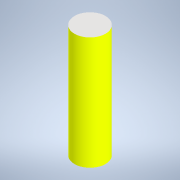
# Autodesk Inventor part: pieza2
Saved by Autodesk Inventor 2021 (Build 250183000, 183)
## iProperties
Created: 2023-05-09
Part Number: pieza2
Material: Generic
Document SubType Name: Modeling
Designer: assman
Density: 1 g/cm^3
Appearance: Default
Author: assman
Autodesk Inventor part; units mm, degrees
ref_plane "YZ Plane" through (0, 0, 0) normal (1, 0, 0) x (0, 1, 0)
ref_plane "XZ Plane" through (0, 0, 0) normal (0, 1, 0) x (-1, 0, 0)
ref_plane "XY Plane" through (0, 0, 0) normal (0, 0, 1) x (1, 0, 0)
sketch "Sketch1" plane through (0, 0, 0) normal (0, 1, 0) x (-1, 0, 0)
  circle A0 centre (0, 0) radius 5.4892
  constraints: 1 centre point, 1 coincident
extrude "Extrusion1" add sketch "Sketch1" along normal blind 40
sketch "Sketch2" plane through (0, 0, 0) normal (0, -1, 0) x (1, 0, 0)
  line L0 (-15.5035, 14.3084) -> (15.5035, 14.3084)
  line L1 (15.5035, 14.3084) -> (15.5035, -14.3084)
  line L2 (15.5035, -14.3084) -> (-15.5035, -14.3084)
  line L3 (-15.5035, -14.3084) -> (-15.5035, 14.3084)
  line L4 (-15.5035, 14.3084) -> (15.5035, -14.3084) construction
  line L5 (15.5035, 14.3084) -> (-15.5035, -14.3084) construction
  point P0 (0, 0)
  constraints: 12 end point, 2 midpoint, 2 parallel, 1 horizontal, 1 perpendicular
extrude "Extrusion2" add sketch "Sketch2" along normal blind 10
body "Solid1"
